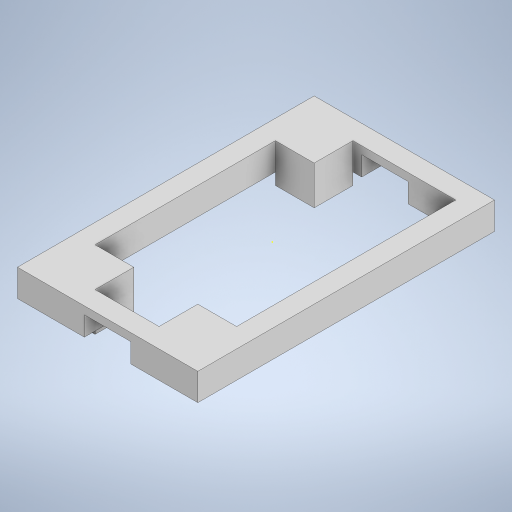
# Autodesk Inventor part: voltage buckboost cover top
Saved by Autodesk Inventor 2024 (Build 280153000, 153)
## iProperties
Created: 2024-06-12
Part Number: voltage buckboost cover top
Material: Generic
Document SubType Name: Modeling
Designer: ony
Density: 1 g/cm^3
Appearance: Default
Author: ony
Autodesk Inventor part; units mm, degrees
ref_plane "YZ Plane" through (0, 0, 0) normal (1, 0, 0) x (0, 1, 0)
ref_plane "XZ Plane" through (0, 0, 0) normal (0, 1, 0) x (-1, 0, 0)
ref_plane "XY Plane" through (0, 0, 0) normal (0, 0, 1) x (1, 0, 0)
sketch "Sketch1" plane through (0, 0, 0) normal (0, 1, 0) x (-1, 0, 0)
  line L0 (25.2467, -36.0292) -> (-21.2533, -36.0292)
  line L1 (-4.0033, -36.0292) -> (-4.0033, -31.0292)
  line L2 (-21.2533, -36.0292) -> (-4.0033, -36.0292)
  line L3 (-4.0033, -36.0292) -> (-4.0033, -31.0292)
  line L4 (-4.0033, -31.0292) -> (-16.2533, -31.0292)
  line L5 (-4.0033, -31.0292) -> (-16.2533, -31.0292)
  line L6 (-16.2533, -31.0292) -> (-16.2533, 35.4708)
  line L7 (-16.2533, -31.0292) -> (-16.2533, 35.4708)
  line L8 (-16.2533, 35.4708) -> (-4.0033, 35.4708)
  line L9 (-4.0033, 35.4708) -> (-4.0033, 40.4708)
  line L10 (-21.2533, 40.4708) -> (25.2467, 40.4708)
  line L11 (-21.2533, -36.0292) -> (-21.2533, 40.4708)
  line L12 (-21.2533, 40.4708) -> (-4.0033, 40.4708)
  line L13 (-21.2533, 40.4708) -> (-21.2533, -36.0292)
  line L14 (7.9967, -31.0292) -> (7.9967, -36.0292)
  line L15 (7.9967, -36.0292) -> (25.2467, -36.0292)
  line L16 (25.2467, -36.0292) -> (25.2467, 40.4708)
  line L17 (25.2467, -36.0292) -> (25.2467, 40.4708)
  line L18 (25.2467, 40.4708) -> (7.9967, 40.4708)
  line L19 (7.9967, 40.4708) -> (7.9967, 35.4708)
  line L20 (7.9967, 35.4708) -> (7.9967, 40.4708)
  line L21 (20.2467, -31.0292) -> (7.9967, -31.0292)
  line L22 (7.9967, -36.0292) -> (7.9967, -31.0292)
  line L23 (7.9967, -31.0292) -> (20.2467, -31.0292)
  line L24 (20.2467, 35.4708) -> (20.2467, -31.0292)
  line L25 (20.2467, -31.0292) -> (20.2467, 35.4708)
  line L26 (7.9967, 35.4708) -> (20.2467, 35.4708)
  line L27 (20.2467, 35.4708) -> (7.9967, 35.4708)
  point P0 (0, 0)
  constraints: 56 end point, 10 collinear, 4 perpendicular, 4 point on line
extrude "Extrusion1" add sketch "Sketch1" along normal blind 5 contours L0 L14 L21 L24 L26 L19 L10 L16 | L0 L11 L10 L9 L8 L6 L4 L1
sketch "Sketch2" plane through (0, 5, 0) normal (0, 1, 0) x (1, 0, 0)
  point P0 (0, 0)
sketch "Sketch3" plane through (0, 5, 0) normal (0, 1, 0) x (1, 0, 0)
  line L0 (-20.2467, -35.4708) -> (-20.2467, 31.0292) projected
  line L1 (-20.2467, -35.4708) -> (-10.2467, -35.4708)
  line L2 (-10.2467, -35.4708) -> (-10.2467, -25.4708)
  line L3 (-10.2467, -25.4708) -> (-20.2467, -25.4708)
  line L4 (-20.2467, -25.4708) -> (-20.2467, -35.4708)
  line L5 (16.2533, 31.0292) -> (16.2533, -35.4708) projected
  line L6 (16.2533, -35.4708) -> (6.2533, -35.4708)
  line L7 (6.2533, -35.4708) -> (6.2533, -25.4708)
  line L8 (6.2533, -25.4708) -> (16.2533, -25.4708)
  line L9 (16.2533, -25.4708) -> (16.2533, -35.4708)
  line L10 (-20.2467, 31.0292) -> (-10.2467, 31.0292)
  line L11 (-10.2467, 31.0292) -> (-10.2467, 21.0292)
  line L12 (-10.2467, 21.0292) -> (-20.2467, 21.0292)
  line L13 (-20.2467, 21.0292) -> (-20.2467, 31.0292)
  point P0 (0, 0)
  dimension "d2" = 10
  dimension "d3" = 10
  dimension "d4" = 10
  dimension "d5" = 10
  dimension "d6" = 10
  dimension "d7" = 10
  constraints: 24 end point, 6 parallel, 3 horizontal, 3 perpendicular
  measures "d2" distance of L3.end L2.end
  measures "d3" distance of L2.end L1.end
  measures "d4" distance of L7.end L8.end
  measures "d5" distance of L6.end L7.end
  measures "d6" distance of L11.end L12.end
  measures "d7" distance of L10.end L11.end
extrude "Extrusion2" add sketch "Sketch3" against normal blind 8
sketch "Sketch4" plane through (0, 5, 0) normal (0, 1, 0) x (1, 0, 0)
  line L0 (-25.2467, 36.0292) -> (-25.2467, -40.4708) projected
  line L1 (21.2533, -40.4708) -> (21.2533, 36.0292) projected
  line L2 (-25.2467, -40.4708) -> (21.2533, -40.4708)
  line L3 (21.2533, -40.4708) -> (21.2533, 36.0292)
  line L4 (21.2533, 36.0292) -> (-25.2467, 36.0292)
  line L5 (-25.2467, 36.0292) -> (-25.2467, -40.4708)
  line L6 (16.2533, 31.0292) -> (16.2533, -25.4708) projected
  line L7 (-20.2467, -35.4708) -> (-20.2467, -25.4708) projected
  line L8 (16.2533, 31.0292) -> (-20.2467, 31.0292)
  line L9 (-20.2467, 31.0292) -> (-20.2467, -35.4708)
  line L10 (-20.2467, -35.4708) -> (16.2533, -35.4708)
  line L11 (16.2533, -35.4708) -> (16.2533, 31.0292)
  point P0 (0, 0)
  constraints: 16 end point, 4 parallel, 2 horizontal, 2 perpendicular
extrude "Extrusion3" add sketch "Sketch4" along normal blind 2
sketch "Sketch5" plane through (0, 5, 0) normal (0, 1, 0) x (1, 0, 0)
  line L0 (-10.2467, -25.4708) -> (-10.2467, -35.4708) projected
  line L1 (-20.2467, -35.4708) -> (-20.2467, -25.4708) projected
  line L2 (-10.2467, -25.4708) -> (-20.2467, -25.4708)
  line L3 (-20.2467, -25.4708) -> (-20.2467, -35.4708)
  line L4 (-20.2467, -35.4708) -> (-10.2467, -35.4708)
  line L5 (-10.2467, -35.4708) -> (-10.2467, -25.4708)
  line L6 (-20.2467, 21.0292) -> (-10.2467, 21.0292) projected
  line L7 (-20.2467, 31.0292) -> (16.2533, 31.0292) projected
  line L8 (-10.2467, 21.0292) -> (-20.2467, 21.0292)
  line L9 (-20.2467, 21.0292) -> (-20.2467, 31.0292)
  line L10 (-20.2467, 31.0292) -> (-10.2467, 31.0292)
  line L11 (-10.2467, 31.0292) -> (-10.2467, 21.0292)
  line L12 (16.2533, -25.4708) -> (6.2533, -25.4708) projected
  line L13 (16.2533, -25.4708) -> (16.2533, -35.4708) projected
  line L14 (6.2533, -25.4708) -> (16.2533, -25.4708)
  line L15 (16.2533, -25.4708) -> (16.2533, -35.4708)
  line L16 (16.2533, -35.4708) -> (6.2533, -35.4708)
  line L17 (6.2533, -35.4708) -> (6.2533, -25.4708)
  point P0 (0, 0)
  constraints: 24 end point, 6 parallel, 3 horizontal, 3 perpendicular
extrude "Extrusion4" add sketch "Sketch5" along normal blind 2
body "Solid1"
